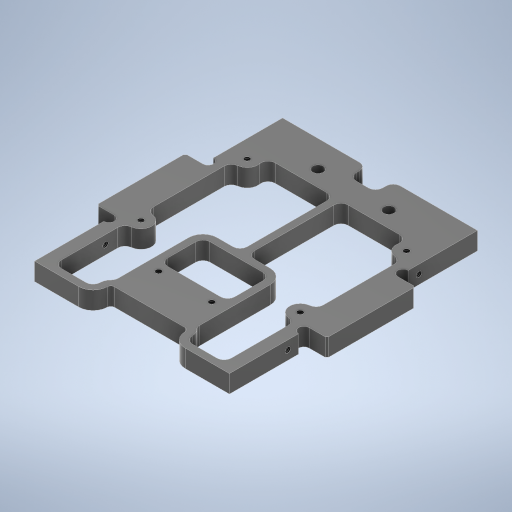
# Autodesk Inventor part: HeadCircuitMountFrame
Saved by Autodesk Inventor 2024.2 (Build 282272000, 272)
## iProperties
Created: 2024-01-19
Part Number: HeadCircuitMountFrame
Material: Acetal Resin, Black
Document SubType Name: Modeling
Designer: Masato Kubotera
Density: 1.425 g/cm^3
Appearance: Smooth - Black
Mass: 11.7532 g
Surface Area: 68.8447 cm^2
Volume: 8.24788 cm^3
Vendor: meviy
Author: Masato Kubotera
Autodesk Inventor part; units mm, degrees
ref_plane "YZ Plane" through (0, 0, 0) normal (1, 0, 0) x (0, 1, 0)
ref_plane "XZ Plane" through (0, 0, 0) normal (0, 1, 0) x (-1, 0, 0)
ref_plane "XY Plane" through (0, 0, 0) normal (0, 0, 1) x (1, 0, 0)
sketch "Sketch1" plane through (0, 0, 0) normal (0, 0, 1) x (1, 0, 0)
  line L0 (35, 27.5) -> (-35, 27.5) construction
  line L1 (-35, 27.5) -> (-35, -27.5) construction
  line L2 (-35, -27.5) -> (35, -27.5) construction
  line L3 (35, -27.5) -> (35, 27.5) construction
  line L4 (35, 27.5) -> (-35, -27.5) construction
  line L5 (-35, 27.5) -> (35, -27.5) construction
  line L6 (0, 27.5) -> (0, -27.5) construction
  line L7 (35, 0) -> (-35, 0) construction
  line L8 (12.5, 27.5) -> (12.5, 32.5)
  line L9 (12.5, 32.5) -> (-12.5, 32.5)
  line L10 (-12.5, 32.5) -> (-12.5, 27.5)
  arc A0 (-15.5, 27.5) -> (-12.5, 27.5) centre (-14, 27.5) ccw
  line L11 (12.5, -27.5) -> (12.5, -32.5)
  line L12 (12.5, -32.5) -> (-12.5, -32.5)
  line L13 (-12.5, -32.5) -> (-12.5, -27.5)
  arc A1 (-12.5, -27.5) -> (-15.5, -27.5) centre (-14, -27.5) ccw
  line L14 (-18.5, 27.5) -> (-18.5, 21.5) construction
  line L15 (0, 32.5) -> (0, 27.5) construction
  line L16 (18.5, 27.5) -> (18.5, 21.5) construction
  arc A2 (12.5, 27.5) -> (15.5, 27.5) centre (14, 27.5) ccw
  arc A3 (15.5, -27.5) -> (12.5, -27.5) centre (14, -27.5) ccw
  line L17 (27.5, -10) -> (5, -10) construction
  line L18 (5, -10) -> (5, 10) construction
  line L19 (5, 10) -> (27.5, 10) construction
  line L20 (27.5, 10) -> (27.5, -10) construction
  line L21 (27.5, -10) -> (5, 10) construction
  line L22 (5, -10) -> (27.5, 10) construction
  line L23 (20, -7.5) -> (20, 7.5) construction
  line L24 (35, -27.5) -> (35, -15)
  line L25 (30, -10) -> (30, 10)
  line L26 (35, 15) -> (35, 27.5)
  arc A4 (31, 11) -> (30, 10) centre (31, 10) ccw
  arc A5 (31, 11) -> (35, 15) centre (31, 15) ccw
  line L27 (-27.5, -10) -> (-27.5, 10) construction
  circle A6 centre (-27.5, 10) radius 2.5 construction
  line L28 (-33, 3.75) -> (-32, 3.75)
  line L29 (-30, 1.75) -> (-30, -1.75)
  line L30 (-32, -3.75) -> (-33, -3.75)
  line L31 (-35, -5.75) -> (-35, -27.5)
  line L32 (-35, 5.75) -> (-35, 27.5)
  arc A7 (-33, -3.75) -> (-35, -5.75) centre (-33, -5.75) ccw
  arc A8 (-32, -3.75) -> (-30, -1.75) centre (-32, -1.75) ccw
  arc A9 (-30, 1.75) -> (-32, 3.75) centre (-32, 1.75) ccw
  arc A10 (-35, 5.75) -> (-33, 3.75) centre (-33, 5.75) ccw
  line L33 (35, -27.5) -> (15.5, -27.5)
  line L34 (-15.5, -27.5) -> (-35, -27.5)
  line L35 (-35, 27.5) -> (-15.5, 27.5)
  line L36 (15.5, 27.5) -> (35, 27.5)
  line L37 (7.5, 9.5) -> (15.5, 9.5)
  line L38 (17.5, 7.5) -> (17.5, -7.5)
  line L39 (15.5, -9.5) -> (7.5, -9.5)
  line L40 (5.5, -7.5) -> (5.5, 7.5)
  line L41 (5.5, 9.5) -> (17.5, -9.5) construction
  line L42 (17.5, 9.5) -> (5.5, -9.5) construction
  circle A11 centre (20, 7.5) radius 2.5 construction
  line L43 (12.5, -25) -> (-22.5, -25) construction
  line L44 (-22.5, -25) -> (-22.5, 25) construction
  line L45 (-22.5, 25) -> (12.5, 25) construction
  line L46 (12.5, 25) -> (12.5, -25) construction
  line L47 (12.5, -25) -> (-22.5, 25) construction
  line L48 (-22.5, -25) -> (12.5, 25) construction
  line L49 (10, 22.5) -> (-20, 22.5) construction
  line L50 (-20, 22.5) -> (-20, -22.5) construction
  line L51 (-20, -22.5) -> (10, -22.5) construction
  line L52 (10, -22.5) -> (10, 22.5) construction
  line L53 (10, 22.5) -> (-20, -22.5) construction
  line L54 (-20, 22.5) -> (10, -22.5) construction
  circle A12 centre (-20, 22.5) radius 2.5 construction
  arc A13 (-20.6, 19.5606) -> (-17.015, 22.2) centre (-20, 22.5) ccw
  line L55 (-23, 17.601) -> (-23, 3)
  line L56 (-15.0251, 24) -> (5.0251, 24)
  arc A14 (7.015, 22.2) -> (12.985, 22.2) centre (10, 22.5) ccw
  arc A15 (31, 13) -> (28.8576, 12.1) centre (31, 10) ccw
  line L57 (33, 15) -> (33, 22)
  line L58 (31, 24) -> (14.9749, 24)
  arc A16 (31, 13) -> (33, 15) centre (31, 15) ccw
  line L59 (35, 15) -> (33, 15) construction
  line L60 (31, 11) -> (31, 13) construction
  line L61 (27.4293, 11.5) -> (7.5, 11.5)
  line L62 (3.5, 7.5) -> (3.5, 3)
  line L63 (1.5, 1) -> (-21, 1)
  arc A17 (27.4293, 11.5) -> (28.8576, 12.1) centre (27.4293, 13.5) ccw
  arc A18 (33, 22) -> (31, 24) centre (31, 22) ccw
  arc A19 (14.9749, 24) -> (12.985, 22.2) centre (14.9749, 22) ccw
  arc A20 (7.015, 22.2) -> (5.0251, 24) centre (5.0251, 22) ccw
  arc A21 (-15.0251, 24) -> (-17.015, 22.2) centre (-15.0251, 22) ccw
  arc A22 (-20.6, 19.5606) -> (-23, 17.601) centre (-21, 17.601) ccw
  arc A23 (-23, 3) -> (-21, 1) centre (-21, 3) ccw
  arc A24 (1.5, 1) -> (3.5, 3) centre (1.5, 3) ccw
  arc A25 (7.5, 11.5) -> (3.5, 7.5) centre (7.5, 7.5) ccw
  arc A26 (30, -10) -> (31, -11) centre (31, -10) ccw
  arc A27 (35, -15) -> (31, -11) centre (31, -15) ccw
  arc A28 (-17.015, -22.2) -> (-20.6, -19.5606) centre (-20, -22.5) ccw
  line L64 (-23, -17.601) -> (-23, -3)
  line L65 (-15.0251, -24) -> (5.0251, -24)
  arc A29 (12.985, -22.2) -> (7.015, -22.2) centre (10, -22.5) ccw
  arc A30 (28.8576, -12.1) -> (31, -13) centre (31, -10) ccw
  line L66 (33, -15) -> (33, -22)
  line L67 (31, -24) -> (14.9749, -24)
  arc A31 (33, -15) -> (31, -13) centre (31, -15) ccw
  line L68 (27.4293, -11.5) -> (7.5, -11.5)
  line L69 (3.5, -7.5) -> (3.5, -3)
  line L70 (1.5, -1) -> (-21, -1)
  arc A32 (28.8576, -12.1) -> (27.4293, -11.5) centre (27.4293, -13.5) ccw
  arc A33 (31, -24) -> (33, -22) centre (31, -22) ccw
  arc A34 (12.985, -22.2) -> (14.9749, -24) centre (14.9749, -22) ccw
  arc A35 (5.0251, -24) -> (7.015, -22.2) centre (5.0251, -22) ccw
  arc A36 (-17.015, -22.2) -> (-15.0251, -24) centre (-15.0251, -22) ccw
  arc A37 (-23, -17.601) -> (-20.6, -19.5606) centre (-21, -17.601) ccw
  arc A38 (-21, -1) -> (-23, -3) centre (-21, -3) ccw
  arc A39 (3.5, -3) -> (1.5, -1) centre (1.5, -3) ccw
  arc A40 (3.5, -7.5) -> (7.5, -11.5) centre (7.5, -7.5) ccw
  arc A41 (15.5, -9.5) -> (17.5, -7.5) centre (15.5, -7.5) ccw
  arc A42 (5.5, -7.5) -> (7.5, -9.5) centre (7.5, -7.5) ccw
  arc A43 (7.5, 9.5) -> (5.5, 7.5) centre (7.5, 7.5) ccw
  arc A44 (17.5, 7.5) -> (15.5, 9.5) centre (15.5, 7.5) ccw
  point P0 (0, 0)
  point P1 (0, 0)
  point P2 (0, -0.0008)
  point P3 (-15.5, -27.5)
  point P4 (12.5, -27.5)
  point P5 (-12.5, -27.5)
  point P6 (-12.5, -27.5)
  point P7 (12.5, -27.5)
  point P8 (16.25, 0)
  point P9 (15.5, -27.5)
  point P10 (11.5, 0)
  point P11 (-5, 0)
  point P12 (-35, -16.625)
  point P13 (-23, 22.5)
  point P14 (-17.4019, 24)
  point P15 (7.4019, 24)
  point P16 (12.5981, 24)
  point P17 (28.4019, 11.5)
  point P18 (30, -9.8466)
  dimension "d19" = 5
  dimension "d20" = 25
  dimension "d37" = 55
  dimension "d40" = 6
  dimension "d41" = 6
  dimension "d59" = 70
  dimension "d60" = 1.5
  dimension "d61" = 22.5
  dimension "d62" = 20
  dimension "d63" = 15
  dimension "d84" = 7.5
  dimension "d87" = 5
  dimension "d88" = 2.5
  dimension "d89" = 32.5
  dimension "d90" = 20
  dimension "d98" = 5
  dimension "d99" = 2
  dimension "d100" = 7.5
  dimension "d101" = 5
  dimension "d109" = 0.5
  dimension "d110" = 0.5
  dimension "d111" = 5
  dimension "d113" = 50
  dimension "d114" = 35
  dimension "d115" = 5
  dimension "d117" = 5
  dimension "d118" = 2
  dimension "d119" = 2
  dimension "d120" = 2
  dimension "d121" = 2
  dimension "d122" = 2
  dimension "d123" = 2
  dimension "d124" = 2
  dimension "d125" = 2
  dimension "d126" = 3
  constraints: 140 end point, 89 point on circle, 51 symmetric about line, 45 centre point, 43 tangent, 19 point on line, 17 midpoint, 16 coincident, 14 equal radius, 13 horizontal, 11 vertical, 10 parallel, 9 collinear, 5 perpendicular, 30 other
  measures "d19" distance of L8.start L8.end
  measures "d20" distance of L8.end L9.end
  measures "d37" distance of L2.end L3.end
  measures "d40" distance of L14.start L14.end
  measures "d41" distance between parallel lines of L10 L14
  measures "d59" distance of L3.end L1.start
  measures "d60" radius of A2
  measures "d61" distance of L18.end L19.end
  measures "d62" distance of L17.end L18.end
  measures "d63" distance of L23.start L23.end
  measures "d84" distance between parallel lines of L20 L23
  measures "d87" distance between parallel lines of L3 L25
  measures "d88" distance between parallel lines of L25 L20
  measures "d89" distance between parallel lines of L18 L27
  measures "d90" distance of L27.start L27.end
  measures "d98" diameter of A6
  measures "d99" radius of A7
  measures "d100" distance between parallel lines of L28 L30
  measures "d101" distance between parallel lines of L29 L1
  measures "d109" distance between parallel lines of L19 L37
  measures "d110" distance between parallel lines of L18 L40
  measures "d111" diameter of A11
  measures "d113" distance of L43.end L44.end
  measures "d114" distance of L43.start L43.end
  measures "d115" distance between parallel lines of L27 L44
  measures "d117" diameter of A12
  measures "d118" distance edge to line of A6 L55
  measures "d119" radius of A16
  measures "d120" radius of A17
  measures "d121" radius of A41
  measures "d122" distance between parallel lines of L61 L37
  measures "d123" radial gap between concentric circles of A15 A4
  measures "d124" distance edge to line of A2 L58
  measures "d125" distance between parallel lines of L63 L70
  measures "d126" radius of A14
extrude "Extrusion1" add sketch "Sketch1" against normal blind 5
hole "M2" at (20, -7.5, 0) at (20, 7.5, 0) at (10, 22.5, 0) at (-20, 22.5, 0) at (-20, -22.5, 0) at (10, -22.5, 0) direction (0, 0, -1) diameter 1.567 end through all thread size "M2x0.4" class "6H" standard "ANSI Metric M Profile"
hole "Phi3" at (-27.5, -10, 0) at (-27.5, 10, 0) direction (0, 0, -1) diameter 3 end through all
sketch "Sketch3" plane through (15.5, 27.5, 0) normal (0, 1, 0) x (1, 0, 0)
  line L0 (19.5, 0) -> (0, 0) projected
  line L1 (3, 0) -> (3, 5)
  line L2 (-31, 0) -> (-50.5, 0) projected
  line L3 (-34, 0) -> (-34, 5)
  line L4 (-50.5, 5) -> (-31, 5) projected
  line L5 (0, 5) -> (19.5, 5) projected
  point P0 (-15.5, 0)
  point P1 (3, 0)
  point P2 (3, 2.5)
  point P3 (-34, 2.5)
  constraints: 4 end point, 2 midpoint, 2 point on line, 2 vertical
hole "Side-M2" at (18.5, 27.5, -2.5) at (-18.5, 27.5, -2.5) direction (0, -1, 0) diameter 1.567 depth 6.3 thread size "M2x0.4" class "6H" standard "ANSI Metric M Profile"
chamfer "Chamfer1" distance 0.5 angle 45 4 edges at (12.5, -32.5, -2.5) (-12.5, -32.5, -2.5) (12.5, 32.5, -2.5) (-12.5, 32.5, -2.5)
mirror "Mirror1" about plane through (0, 0, 0) normal (0, 1, 0) of "Side-M2"
body "Solid1"
